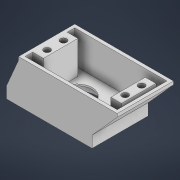
# Autodesk Inventor part: Übersetzungsbox_2
Saved by Autodesk Inventor 2021 (Build 250183000, 183)
## iProperties
Created: 2021-01-10
Part Number: Übersetzungsbox_2
Material: Generisch
Document SubType Name: Modeling
Designer: Ctroi
Density: 1 g/cm^3
Appearance: Vorgabe
Author: Ctroi
## iProperties of the stored document _3D-Druck.ipt
Created: 2021-01-13
Part Number: _3D-Druck
Material: Generisch
Document SubType Name: Modeling
Designer: Ctroi
Density: 1 g/cm^3
Appearance: Vorgabe
Author: Ctroi
Autodesk Inventor part; units mm, degrees
ref_plane "YZ Plane" through (0, 0, 0) normal (1, 0, 0) x (0, 1, 0)
ref_plane "XZ Plane" through (0, 0, 0) normal (0, 1, 0) x (-1, 0, 0)
ref_plane "XY Plane" through (0, 0, 0) normal (0, 0, 1) x (1, 0, 0)
sketch "Skizze1" plane through (0, 0, 0) normal (0, 1, 0) x (-1, 0, 0)
  line L0 (-26, -17.1) -> (26, -17.1)
  line L1 (26, -17.1) -> (26, 17.1)
  line L2 (26, 17.1) -> (-26, 17.1)
  line L3 (-26, 17.1) -> (-26, -17.1)
  line L4 (0, -23.94) -> (0, 23.94) projected
  line L5 (-36.4, 0) -> (36.4, 0) projected
  point P0 (0, 0)
  dimension "d0" = 52
  dimension "d1" = 34.2
  constraints: 8 end point, 2 parallel, 1 horizontal, 1 perpendicular, 2 other
  measures "d0" distance of L1.end L2.end
  measures "d1" distance of L0.end L1.end
extrude "Extrusion1" add sketch "Skizze1" along normal blind 7
ref_plane "Arbeitsebene1" through (0, 24, 0) normal (0, 1, 0) x (1, 0, 0)
sketch "Skizze2" plane through (0, 24, 0) normal (0, 1, 0) x (1, 0, 0)
  line L0 (26, 17.1) -> (-26, 17.1) projected
  line L1 (-18.7, 17.1) -> (41.3, 17.1)
  line L2 (41.3, 17.1) -> (41.3, -17.1)
  line L3 (41.3, -17.1) -> (-18.7, -17.1)
  line L4 (-18.7, -17.1) -> (-18.7, 17.1)
  line L5 (-26, 17.1) -> (-26, -17.1) projected
  point P0 (0, 0)
  dimension "d5" = 60
  dimension "d6" = 34.2
  dimension "d7" = 7.3
  constraints: 8 end point, 2 parallel, 1 horizontal, 1 perpendicular, 1 point on line
  measures "d5" distance of L2.end L3.end
  measures "d6" distance of L1.end L2.end
  measures "d7" distance between parallel lines of L5 L4
extrude "Extrusion2" add sketch "Skizze2" along normal blind 2
loft "Erhebung1" add section 1 edges at (-26, 7, 0) (0, 7, 17.1) (26, 7, 0) (0, 7, -17.1) section 2 edges at (41.3, 24, 0) (11.3, 24, 17.1) (-18.7, 24, 0) (11.3, 24, -17.1)
shell "Wandung1" thickness 2 removed faces 1 at (21.3, 26, -5.7)
sketch "Skizze7" plane through (-24, 2, 15.1) normal (0, 1, 0) x (1, 0, 0)
  line L0 (-2, 32.2) -> (-2, -2) projected
  line L1 (50, 32.2) -> (-2, 32.2) projected
  line L2 (-2, -2) -> (50, -2)
  line L3 (50, -2) -> (50, 32.2)
  line L4 (50, 32.2) -> (-2, 32.2)
  line L5 (-2, 32.2) -> (-2, -2)
  line L6 (48, 0) -> (0, 0)
  line L7 (0, 0) -> (0, 30.2)
  line L8 (0, 30.2) -> (48, 30.2)
  line L9 (48, 30.2) -> (48, 0)
  point P0 (24, 15.1)
  dimension "d28" = 2
  constraints: 16 end point, 4 parallel, 2 perpendicular, 1 horizontal, 3 other
  measures "d28" distance between parallel lines of L2 L6
extrude "Extrusion5" add sketch "Skizze7" along normal blind 4 contours L6 L7 L8 L9
sketch "Skizze11" plane through (0, 26, 0) normal (0, 1, 0) x (1, 0, 0)
  line L0 (-16.7, -15.1) -> (-16.7, 15.1) projected
  line L1 (-16.7, 10.5) -> (-10.2, 10.5)
  line L2 (-10.2, 10.5) -> (-10.2, -10.5)
  line L3 (-10.2, -10.5) -> (-16.7, -10.5)
  line L4 (-16.7, -10.5) -> (-16.7, 10.5)
  line L5 (54.76, 0) -> (-39.46, 0) projected
  line L6 (37.3, -10.5) -> (30.8, -10.5)
  line L7 (30.8, -10.5) -> (30.8, 10.5)
  line L8 (30.8, 10.5) -> (37.3, 10.5)
  line L9 (37.3, 10.5) -> (37.3, -10.5)
  line L10 (41.3, -17.1) -> (41.3, 17.1) projected
  line L11 (-18.7, 17.1) -> (-18.7, -17.1) projected
  point P0 (0, 0)
  dimension "d49" = 6.5
  dimension "d50" = 21
  dimension "d58" = 6.5
  dimension "d59" = 21
  dimension "d87" = 10.5
  dimension "d88" = 8.5
  constraints: 16 end point, 3 parallel, 2 horizontal, 1 perpendicular, 1 point on line, 2 other
  measures "d49" distance of L2.end L3.end
  measures "d50" distance of L1.end L2.end
  measures "d58" distance of L7.end L8.end
  measures "d59" distance of L6.end L7.end
  measures "d87" distance between parallel lines of L10 L7
  measures "d88" distance between parallel lines of L11 L2
extrude "Extrusion9" add sketch "Skizze11" against normal blind 6 contours L0 L5 L2 L3 | L0 L1 L2 L5
thicken "Verdickung1" operation add thickness 1 both sides no extend neighbours yes toward (-1, 0, 0) faces at (-16.7, 22.3925, -3.5) (-21.5667, 12.2554, 3.5)
extrude "Extrusion11" add sketch "Skizze11" against normal blind 12 contours L9 L6 L7 L5 | L5 L7 L8 L9
sketch "Skizze13" plane through (0, 26, 0) normal (0, 1, 0) x (1, 0, 0)
  circle A0 centre (-13.45, 5) radius 1.95
  line L0 (-10.2, -10.5) -> (-10.2, 10.5) projected
  circle A1 centre (-13.45, -5) radius 1.95
  line L1 (54.76, 0) -> (-39.46, 0) projected
  circle A2 centre (34.05, 5) radius 1.95
  line L2 (30.8, 10.5) -> (30.8, -10.5) projected
  circle A3 centre (34.05, -5) radius 1.95
  point P0 (0, 0)
  dimension "d65" = 3.9
  dimension "d66" = 3.25
  dimension "d67" = 3.9
  dimension "d68" = 5
  dimension "d69" = 5
  dimension "d70" = 3.25
  dimension "d71" = 3.9
  dimension "d72" = 3.25
  dimension "d73" = 5
  dimension "d74" = 3.9
  dimension "d75" = 3.25
  dimension "d76" = 5
  constraints: 4 centre point
  measures "d65" diameter of A0
  measures "d66" distance from line of L0 A0.centre
  measures "d67" diameter of A1
  measures "d68" distance from line of L1 A0.centre
  measures "d69" distance from line of L1 A1.centre
  measures "d70" distance from line of L0 A1.centre
  measures "d71" diameter of A2
  measures "d72" distance from line of L2 A2.centre
  measures "d73" distance from line of L1 A2.centre
  measures "d74" diameter of A3
  measures "d75" distance from line of L2 A3.centre
  measures "d76" distance from line of L1 A3.centre
extrude "Extrusion12" cut sketch "Skizze13" against normal blind 5.7
sketch "Skizze14" plane through (0, 20, 0) normal (0, -1, 0) x (1, 0, 0)
  line L0 (-10.2, 10.5) -> (-10.2, -10.5) projected
  line L1 (-17.1528, -10.5) -> (-16.7, -10.5) projected
  line L2 (-10.2, 10.5) -> (-16.7, 10.5)
  line L3 (-16.7, 10.5) -> (-16.7, -10.5)
  line L4 (-16.7, -10.5) -> (-10.2, -10.5)
  line L5 (-10.2, -10.5) -> (-10.2, 10.5)
  point P0 (0, 0)
  constraints: 8 end point, 2 parallel, 1 horizontal, 1 perpendicular
extrude "Extrusion13" add sketch "Skizze14" along normal up to surface (14 mm away)
sketch "Skizze15" plane through (0, 0, 0) normal (0, -1, 0) x (1, 0, 0)
  circle A0 centre (0, 0) radius 12.1
  dimension "d81" = 24.2
  constraints: 1 centre point, 1 coincident
  measures "d81" diameter of A0
extrude "Extrusion14" cut sketch "Skizze15" against normal blind 5
sketch "Skizze16" plane through (0, 5, 0) normal (0, -1, 0) x (1, 0, 0)
  circle A0 centre (0, 0) radius 9
  dimension "d84" = 18
  constraints: 1 centre point, 1 coincident
  measures "d84" diameter of A0
extrude "Extrusion15" cut sketch "Skizze16" against normal up to surface (1 mm away)
sketch "Skizze19" plane through (32.3, 14, 10.5) normal (0, 0, 1) x (1, 0, 0)
  line L0 (5, 0) -> (5, 5.5556)
  line L1 (-6.3, -7) -> (9, 10) projected
  line L2 (5, 0) -> (0, 0) projected
  line L3 (5, 5.5556) -> (5, 0) projected
  line L4 (0, 0) -> (5, 0)
  point P0 (-32.3, -14)
  constraints: 4 end point, 1 perpendicular, 1 point on line, 1 vertical
extrude "Extrusion18" cut sketch "Skizze19" against normal up to surface (21 mm away)
sketch "Skizze17" plane through (-26, 0, 17.1) normal (0, 0, 1) x (1, 0, 0)
  line L0 (18.3, 23) -> (34, 23)
  line L1 (34, 23) -> (34, 7)
  line L2 (34, 7) -> (18.3, 7)
  line L3 (18.3, 7) -> (18.3, 23)
  line L4 (7.3, 26) -> (67.3, 26) projected
  line L5 (7.3, 24) -> (7.3, 26) projected
  line L6 (0, 0) -> (52, 0) projected
  line L7 (52, 0) -> (52, 7) projected
  point P0 (26, 0)
  dimension "d97" = 3
  dimension "d98" = 11
  dimension "d99" = 7
  dimension "d100" = 18
  constraints: 8 end point, 2 parallel, 1 horizontal, 1 perpendicular
  measures "d97" distance between parallel lines of L4 L0
  measures "d98" distance between parallel lines of L5 L3
  measures "d99" distance between parallel lines of L6 L2
  measures "d100" distance between parallel lines of L7 L1
sketch "Skizze18" plane through (26, 0, -17.1) normal (0, 0, -1) x (-1, 0, 0)
  line L0 (33.7, 23) -> (33.7, 7) projected
  line L1 (2, 6) -> (49.1645, 6) projected
  line L2 (33.7, 23) -> (18, 23)
  line L3 (18, 23) -> (18, 6)
  line L4 (18, 6) -> (33.7, 6)
  line L5 (33.7, 6) -> (33.7, 23)
  line L6 (44.7, 24) -> (44.7, 26) projected
  line L7 (0, 0) -> (0, 7) projected
  point P0 (26, 0)
  dimension "d101" = 11
  dimension "d102" = 18
  constraints: 8 end point, 2 parallel, 1 horizontal, 1 perpendicular, 1 point on line
  measures "d101" distance between parallel lines of L6 L0
  measures "d102" distance between parallel lines of L7 L3
